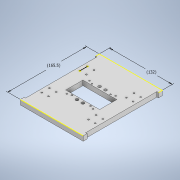
# Autodesk Inventor part: maze_01_test
Saved by Autodesk Inventor 2020 (Build 240168000, 168)
## iProperties
Created: 2022-07-17
Part Number: maze_01_test
Material: Типовые
Document SubType Name: Modeling
Designer: akapu
Density: 1 g/cm^3
Appearance: По умолчанию
Author: akapu
Autodesk Inventor part; units mm, degrees
ref_plane "YZ Plane" through (0, 0, 0) normal (1, 0, 0) x (0, 1, 0)
ref_plane "XZ Plane" through (0, 0, 0) normal (0, 1, 0) x (-1, 0, 0)
ref_plane "XY Plane" through (0, 0, 0) normal (0, 0, 1) x (1, 0, 0)
sketch "Эскиз1" plane through (0, 0, 0) normal (0, 1, 0) x (-1, 0, 0)
  line L0 (0, 0) -> (-132, 0)
  line L1 (-132, -165.5) -> (0, -165.5)
  line L2 (0, -165.5) -> (0, -157.5)
  line L3 (0, -157.5) -> (-3, -157.5)
  line L4 (0, 0) -> (0, -8)
  line L5 (0, -8) -> (-3, -8)
  line L6 (-3, -8) -> (-3, -157.5)
  line L7 (-132, -165.5) -> (-132, -157.5)
  line L8 (-132, -157.5) -> (-129, -157.5)
  line L9 (-129, -157.5) -> (-129, -8)
  line L10 (-129, -8) -> (-132, -8)
  line L11 (-132, -8) -> (-132, 0)
  line L12 (-30.5, -100.75) -> (-101.5, -100.75)
  line L13 (-101.5, -100.75) -> (-101.5, -64.75)
  line L14 (-101.5, -64.75) -> (-30.5, -64.75)
  line L15 (-30.5, -64.75) -> (-30.5, -100.75)
  circle A0 centre (-59.8, -59) radius 3
  circle A1 centre (-72.2, -59) radius 3
  circle A2 centre (-85.5, -61.8) radius 1.5
  circle A3 centre (-93.5, -59) radius 1.5
  circle A4 centre (-93.5, -106.5) radius 1.5
  circle A5 centre (-85.5, -103.7) radius 1.5
  circle A6 centre (-72.2, -106.5) radius 3
  circle A7 centre (-59.8, -106.5) radius 3
  circle A8 centre (-46.5, -103.7) radius 1.5
  circle A9 centre (-38.5, -106.5) radius 1.5
  circle A10 centre (-38.5, -59) radius 1.5
  circle A11 centre (-46.5, -61.8) radius 1.5
  circle A12 centre (-10, -35) radius 1.5
  circle A13 centre (-10, -51) radius 1.5
  circle A14 centre (-24, -51) radius 1.5
  circle A15 centre (-24, -35) radius 1.5
  circle A16 centre (-24, -114.5) radius 1.5
  circle A17 centre (-10, -114.5) radius 1.5
  circle A18 centre (-10, -130.5) radius 1.5
  circle A19 centre (-24, -130.5) radius 1.5
  circle A20 centre (-108, -130.5) radius 1.5
  circle A21 centre (-108, -114.5) radius 1.5
  circle A22 centre (-122, -114.5) radius 1.5
  circle A23 centre (-122, -130.5) radius 1.5
  circle A24 centre (-122, -51) radius 1.5
  circle A25 centre (-108, -51) radius 1.5
  circle A26 centre (-108, -35) radius 1.5
  circle A27 centre (-122, -35) radius 1.5
  constraints: 32 end point, 28 centre point, 3 parallel, 3 perpendicular, 2 horizontal, 2 point on line, 1 vertical
extrude "Выдавливание1" add sketch "Эскиз1" along normal blind 10
sketch "Эскиз2" plane through (0, 10, 0) normal (0, 1, 0) x (1, 0, 0)
  line L0 (132, 157.5) -> (132, 165.5) projected
  line L1 (0, 165.5) -> (0, 157.5) projected
  line L2 (0, 0) -> (132, 0) projected
  line L3 (132, 165.5) -> (0, 165.5) projected
  circle A0 centre (10, 114.5) radius 1.5 projected
  circle A1 centre (10, 130.5) radius 1.5 projected
  line L4 (10, 114.5) -> (10, 130.5)
  dimension "d59" = 132
  dimension "d60" = 165.5
  constraints: 2 end point, 1 vertical
  measures "d59" distance between parallel lines of L0 L1
  measures "d60" distance between parallel lines of L2 L3
